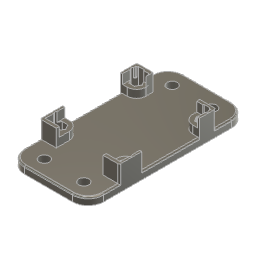
u2d2_mount (Autodesk Fusion 360 design; units mm, degrees)
Autodesk Fusion 360 part; units mm, degrees
sketch "Sketch1" plane through (0, 0, 0) normal (0, 1, 0) x (1, 0, 0)
  line L0 (0, 0) -> (42.469, 0) construction
  line L1 (0, 0) -> (0, 48.4717) construction
  line L2 (25.4, 51.0635) -> (-25.4, 51.0635)
  line L3 (-25.4, 51.0635) -> (-25.4, -51.0635)
  line L4 (-25.4, -51.0635) -> (25.4, -51.0635)
  line L5 (25.4, -51.0635) -> (25.4, 51.0635)
  line L6 (25.4, 51.0635) -> (-25.4, -51.0635) construction
  line L7 (-25.4, 51.0635) -> (25.4, -51.0635) construction
  line L8 (24.0635, 29.0635) -> (-24.0635, 29.0635)
  line L9 (-24.0635, 29.0635) -> (-24.0635, -29.0635)
  line L10 (-24.0635, -29.0635) -> (24.0635, -29.0635)
  line L11 (24.0635, -29.0635) -> (24.0635, 29.0635)
  line L12 (24.0635, 29.0635) -> (-24.0635, -29.0635) construction
  line L13 (-24.0635, 29.0635) -> (24.0635, -29.0635) construction
  circle A0 centre (-21.0635, 26.5635) radius 3.127 construction
  line L14 (-21.0635, 29.6905) -> (-19.2581, 29.6905)
  line L15 (-21.0635, 26.5635) -> (-21.0635, 33) construction
  line L16 (-21.0635, 29.6905) -> (-22.8689, 29.6905)
  line L17 (-23.7716, 28.127) -> (-22.8689, 29.6905)
  line L18 (-23.7716, 28.127) -> (-24.6742, 26.5635)
  line L19 (-23.7716, 25) -> (-24.6742, 26.5635)
  line L20 (-23.7716, 25) -> (-22.8689, 23.4365)
  line L21 (-21.0635, 23.4365) -> (-22.8689, 23.4365)
  line L22 (-21.0635, 23.4365) -> (-19.2581, 23.4365)
  line L23 (-18.3554, 25) -> (-19.2581, 23.4365)
  line L24 (-18.3554, 25) -> (-17.4528, 26.5635)
  line L25 (-18.3554, 28.127) -> (-17.4528, 26.5635)
  line L26 (-18.3554, 28.127) -> (-19.2581, 29.6905)
  line L27 (-25.4, 31.0635) -> (25.4, 31.0635)
  line L28 (-24, 2) -> (-9, 2) construction
  line L29 (18.3554, 28.127) -> (17.4528, 26.5635)
  line L30 (18.3554, 28.127) -> (19.2581, 29.6905)
  line L31 (21.0635, 29.6905) -> (19.2581, 29.6905)
  line L32 (21.0635, 29.6905) -> (22.8689, 29.6905)
  line L33 (23.7716, 28.127) -> (22.8689, 29.6905)
  line L34 (23.7716, 28.127) -> (24.6742, 26.5635)
  line L35 (23.7716, 25) -> (24.6742, 26.5635)
  line L36 (23.7716, 25) -> (22.8689, 23.4365)
  line L37 (21.0635, 23.4365) -> (22.8689, 23.4365)
  line L38 (21.0635, 23.4365) -> (19.2581, 23.4365)
  line L39 (18.3554, 25) -> (19.2581, 23.4365)
  line L40 (18.3554, 25) -> (17.4528, 26.5635)
  line L41 (-21.0635, -25.6905) -> (-19.2581, -25.6905)
  line L42 (-21.0635, -25.6905) -> (-22.8689, -25.6905)
  line L43 (-23.7716, -24.127) -> (-22.8689, -25.6905)
  line L44 (-23.7716, -24.127) -> (-24.6742, -22.5635)
  line L45 (-23.7716, -21) -> (-24.6742, -22.5635)
  line L46 (-23.7716, -21) -> (-22.8689, -19.4365)
  line L47 (-21.0635, -19.4365) -> (-22.8689, -19.4365)
  line L48 (-21.0635, -19.4365) -> (-19.2581, -19.4365)
  line L49 (-18.3554, -21) -> (-19.2581, -19.4365)
  line L50 (-18.3554, -21) -> (-17.4528, -22.5635)
  line L51 (-18.3554, -24.127) -> (-17.4528, -22.5635)
  line L52 (-18.3554, -24.127) -> (-19.2581, -25.6905)
  line L53 (21.0635, -25.6905) -> (19.2581, -25.6905)
  line L54 (21.0635, -25.6905) -> (22.8689, -25.6905)
  line L55 (23.7716, -24.127) -> (22.8689, -25.6905)
  line L56 (23.7716, -24.127) -> (24.6742, -22.5635)
  line L57 (23.7716, -21) -> (24.6742, -22.5635)
  line L58 (23.7716, -21) -> (22.8689, -19.4365)
  line L59 (21.0635, -19.4365) -> (22.8689, -19.4365)
  line L60 (21.0635, -19.4365) -> (19.2581, -19.4365)
  line L61 (18.3554, -21) -> (19.2581, -19.4365)
  line L62 (18.3554, -21) -> (17.4528, -22.5635)
  line L63 (18.3554, -24.127) -> (17.4528, -22.5635)
  line L64 (18.3554, -24.127) -> (19.2581, -25.6905)
  line L65 (-25.4, -31.0635) -> (25.4, -31.0635)
  circle A1 centre (-12.7, 41.0635) radius 3.3
  circle A2 centre (12.7, 41.0635) radius 3.3
  circle A3 centre (12.7, -41.0635) radius 3.3
  circle A4 centre (-12.7, -41.0635) radius 3.3
  circle A5 centre (-21.0635, 26.5635) radius 6
  line L66 (-21.0635, 20.5635) -> (-25.4, 20.5635)
  line L67 (-15.0635, 26.5635) -> (-15.0635, 31.0635)
  line L68 (21.0635, 20.5635) -> (25.4, 20.5635)
  circle A6 centre (21.0635, 26.5635) radius 6
  line L69 (15.0635, 26.5635) -> (15.0635, 31.0635)
  circle A7 centre (21.0635, -22.5635) radius 6
  line L70 (15.0635, -22.5635) -> (15.0635, -27.0635)
  line L71 (21.0635, -16.5635) -> (25.4, -16.5635)
  circle A8 centre (-21.0635, -22.5635) radius 6
  line L72 (-21.0635, -16.5635) -> (-25.4, -16.5635)
  line L73 (-15.0635, -22.5635) -> (-15.0635, -27.0635)
  line L74 (-15.0635, -27.0635) -> (-15.0635, -31.0635)
  line L75 (15.0635, -27.0635) -> (15.0635, -31.0635)
  point P0 (-21.0635, 26.5635)
  point P1 (-21.0635, -22.5635)
  dimension "d24" = 50.8
  dimension "d26" = 58.127
  dimension "d27" = 48.127
  dimension "d28" = 3
  dimension "d29" = 2.5
  dimension "d30" = 6.254
  dimension "d32" = 360
  dimension "d33" = 6.5
  dimension "d34" = 2
  dimension "d35" = 6.6
  dimension "d36" = 12.7
  dimension "d37" = 10
  dimension "d38" = 10
  dimension "d41" = 12
  constraint coincident L0.start L1.start
  constraint horizontal L0
  constraint perpendicular L0 L1
  constraint horizontal L2
  constraint perpendicular L2 L3
  constraint parallel L2 L4
  constraint parallel L3 L5
  constraint coincident L6 L0.start
  constraint coincident L7 L0.start
  constraint horizontal L8
  constraint perpendicular L8 L9
  constraint parallel L8 L10
  constraint parallel L9 L11
  constraint coincident L12 L0.start
  constraint coincident L13 L0.start
  constraint coincident P0 A0.centre
  constraint coincident A0 L14.start
  constraint parallel L8 L14
  constraint vertical L15
  constraint coincident L14.start L15
  constraint symmetric L14.start L15 L16.start
  constraint symmetric L14.end L15 L16.end
  constraint coincident L24.end L25.end
  constraint coincident L3 L27.start
  constraint coincident L5 L27.end
  constraint perpendicular L5 L27
  constraint horizontal L28
  constraint symmetric L1 L14.start L31.start
  constraint symmetric L1 L14.end L30.end
  constraint symmetric L1 L16.end L32.end
  constraint symmetric L1 L17.start L33.start
  constraint symmetric L1 L18.end L34.end
  constraint symmetric L1 L19.start L35.start
  constraint symmetric L1 L20.end L36.end
  constraint symmetric L1 L21.start L37.start
  constraint symmetric L1 L22.end L38.end
  constraint symmetric L1 L23.start L39.start
  constraint symmetric L1 L24.end L29.end
  constraint symmetric L1 L25.start L29.start
  constraint symmetric P0 L28 P1
  constraint symmetric L14.start L28 L41.start
  constraint symmetric L14.end L28 L41.end
  constraint symmetric L16.end L28 L42.end
  constraint symmetric L17.start L28 L43.start
  constraint symmetric L18.end L28 L44.end
  constraint symmetric L19.start L28 L45.start
  constraint symmetric L20.end L28 L46.end
  constraint symmetric L21.start L28 L47.start
  constraint symmetric L22.end L28 L48.end
  constraint symmetric L23.start L28 L49.start
  constraint symmetric L24.end L28 L50.end
  constraint symmetric L25.start L28 L51.start
  constraint symmetric L28 L29.start L63.start
  constraint symmetric L28 L29.end L62.end
  constraint symmetric L28 L30.end L53.end
  constraint symmetric L28 L31.start L53.start
  constraint symmetric L28 L32.end L54.end
  constraint symmetric L28 L33.start L55.start
  constraint symmetric L28 L34.end L56.end
  constraint symmetric L28 L35.start L57.start
  constraint symmetric L28 L36.end L58.end
  constraint symmetric L28 L37.start L59.start
  constraint symmetric L28 L38.end L60.end
  constraint symmetric L28 L39.start L61.start
  constraint symmetric L0 L27.start L65.start
  constraint symmetric L0 L27.end L65.end
  constraint symmetric L1 A1 A2
  constraint symmetric L0 A1 A4
  constraint symmetric L0 A2 A3
  constraint coincident A5 L66.start
  constraint coincident L3 L66.end
  constraint perpendicular L3 L66
  constraint coincident A5 L67.start
  constraint coincident L27 L67.end
  constraint perpendicular L27 L67
  constraint tangent A5 L67
  constraint tangent A5 L66
  constraint symmetric L1 A5 A6
  constraint symmetric L1 L66.start L68.start
  constraint symmetric L1 L66.end L68.end
  constraint symmetric L1 L67.start L69.start
  constraint symmetric L1 L67.end L69.end
  constraint symmetric L28 A5 A8
  constraint symmetric L28 L66.start L72.start
  constraint symmetric L28 L66.end L72.end
  constraint symmetric L28 L67.start L73.start
  constraint symmetric L28 L67.end L73.end
  constraint symmetric L28 L68.start L71.start
  constraint symmetric L28 L68.end L71.end
  constraint symmetric L28 A6 A7
  constraint symmetric L28 L69.start L70.start
  constraint symmetric L28 L69.end L70.end
  constraint coincident L65 L74.end
  constraint perpendicular L65 L74
  constraint symmetric L1 L73.end L70.end
  constraint symmetric L1 L74.end L75.end
  measures "d24" distance of L2.start L2.end
  measures "d26" distance of L8.end L9.end
  measures "d27" distance of L8.start L8.end
  measures "d28" distance of L9 P0
  measures "d29" distance of L8 P0
  measures "d30" diameter of A0
  measures "d33" distance of L10 P1
  measures "d34" distance of L8 L27
  measures "d35" diameter of A1
  measures "d36" distance of L1 A1.centre
  measures "d37" distance of L27 A1.centre
  measures "d38" distance of L2 A1.centre
  measures "d41" diameter of A5
extrude "Extrude1" add sketch "Sketch1" against normal blind 4.7625 contours L2 L3 L5 L27 A5 A6 | L5 L27 A6 | L3 L27 A5 | L5 L8 L11 L27 L30 L31 L32 L33 L34 L35 A6 | L27 A6 | L3 L8 L9 L14 L16 L17 L18 L19 L26 L27 A5 | L27 A5 | L5 L11 L68 A6 | L8 L27 A6 L69 | L3 L9 A5 L66 | L8 L27 A5 L67 | L5 L11 L68 L71 | L8 L11 L29 L30 L35 L36 L37 L38 L39 L40 A6 | L11 L68 A6 | L8 L27 L67 L69 | L8 A6 L69 | L3 L9 L66 L72 | L9 A5 L66 | L8 L9 L19 L20 L21 L22 L23 L24 L25 L26 A5 | L8 A5 L67 | L5 L11 A7 L71 | L8 L9 L10 L11 A5 L66 L67 L68 A6 L69 A7 L70 L71 A8 L72 L73 L74 L75 | L8 L11 L29 L30 L33 L34 L35 L36 L37 L38 L39 L40 | L11 L34 L35 | L8 L30 L31 L32 L33 | L3 L9 A8 L72 | L9 L18 L19 | L8 L9 L17 L18 L19 L20 L21 L22 L23 L24 L25 L26 | L8 L14 L16 L17 L26 | L5 L11 L56 L57 A7 | L11 A7 L71 | L8 L11 L33 L34 | L3 L9 L44 L45 A8 | L9 A8 L72 | L8 L9 L17 L18 | L5 L10 L11 L65 A7 L75 | L11 L53 L54 L55 L56 L57 L58 L59 L60 L61 L62 L63 L64 A7 | L3 L9 L10 L65 A8 L74 | L9 L41 L42 L43 L44 L45 L46 L47 L48 L49 L50 L51 L52 A8 | L3 L4 L5 L65 | L10 L11 A7 L70 L75 | L11 L56 L57 | L11 L53 L54 L55 L56 L57 L58 L59 L60 L61 L62 L63 L64 | L9 L10 A8 L73 L74 | L9 L41 L42 L43 L44 L45 L46 L47 L48 L49 L50 L51 L52 | L9 L44 L45 | L10 L65 L74 L75
extrude "Extrude2" add sketch "Sketch1" along normal blind 5 contours L5 L27 A6 | L3 L27 A5 | L5 L8 L11 L27 L30 L31 L32 L33 L34 L35 A6 | L3 L8 L9 L14 L16 L17 L18 L19 L26 L27 A5 | L5 L11 L68 A6 | L8 L27 A6 L69 | L3 L9 A5 L66 | L8 L27 A5 L67 | L8 L11 L29 L30 L35 L36 L37 L38 L39 L40 A6 | L11 L68 A6 | L8 A6 L69 | L9 A5 L66 | L8 L9 L19 L20 L21 L22 L23 L24 L25 L26 A5 | L8 A5 L67 | L5 L11 A7 L71 | L3 L9 A8 L72 | L5 L11 L56 L57 A7 | L11 A7 L71 | L8 L11 L33 L34 | L3 L9 L44 L45 A8 | L9 A8 L72 | L8 L9 L17 L18 | L5 L10 L11 L65 A7 L75 | L11 L53 L54 L55 L56 L57 L58 L59 L60 L61 L62 L63 L64 A7 | L3 L9 L10 L65 A8 L74 | L9 L41 L42 L43 L44 L45 L46 L47 L48 L49 L50 L51 L52 A8 | L10 L11 A7 L70 L75 | L9 L10 A8 L73 L74
extrude "Extrude3" add sketch "Sketch1" along normal blind 11 contours L5 L27 A6 | L3 L27 A5 | L5 L8 L11 L27 L30 L31 L32 L33 L34 L35 A6 | L3 L8 L9 L14 L16 L17 L18 L19 L26 L27 A5 | L5 L11 L68 A6 | L8 L27 A6 L69 | L3 L9 A5 L66 | L8 L27 A5 L67 | L8 A5 L67 | L5 L11 A7 L71 | L3 L9 A8 L72 | L5 L11 L56 L57 A7 | L3 L9 L44 L45 A8 | L5 L10 L11 L65 A7 L75 | L3 L9 L10 L65 A8 L74
fillet "Fillet1" radius 10 4 edges at (-25.4, -2.3813, 51.0635) (25.4, -2.3813, 51.0635) (-25.4, -2.3813, -51.0635) (25.4, -2.3813, -51.0635)
fillet "Fillet2" radius 1 12 edges at (-25.4, 0, 36.0635) (-22.4711, 0, 48.1346) (0, 0, 51.0635) (22.4711, 0, 48.1346) (25.4, 0, 36.0635) (25.4, 0, -2) (-25.4, 0, -2) (-25.4, 0, -36.0635) (-22.4711, 0, -48.1346) (0, 0, -51.0635) (22.4711, 0, -48.1346) (25.4, 0, -36.0635)
fillet "Fillet3" radius 1 4 edges at (25.4, 5, -31.0635) (25.4, 5, 31.0635) (-25.4, 5, 31.0635) (-25.4, 5, -31.0635)
equation "fitNormal = 0.254 mm"
equation "fitLoose = 0.508 mm"
equation "fitTight = 0.127 mm"
equation "axleToTop = 9.5 mm"
equation "xl330Height = 34 mm"
equation "axletoBottom = xl330Height - axleToTop"
equation "axleDiameter = 16 mm"
equation "boltDiameter = 1.6 mm"
equation "xl330Width = 20 mm"
equation "xl330Length = 23 mm"
equation "l2x = 30 mm"
equation "l3x = 157 mm"
equation "l3y = 9 mm"
equation "baseMount = 10 mm"
equation "l4x = -2 mm + axleToTop + 30 mm + xl330Length"
equation "l4y = 32 mm"
equation "axleDepth = 3 mm"
equation "capOuterWidth = 30 mm"
equation "capHeight = 25 mm"
equation "jcBracketHeight = 8.2 mm"
equation "jcBracketLength = 97.307 mm"
equation "jcWidth = 34 mm"
equation "capToTop = 40 mm"
equation "d26 = 58 mm + fitTight"
equation "d27 = 48 mm + fitTight"
equation "d30 = 6 mm + fitNormal"
